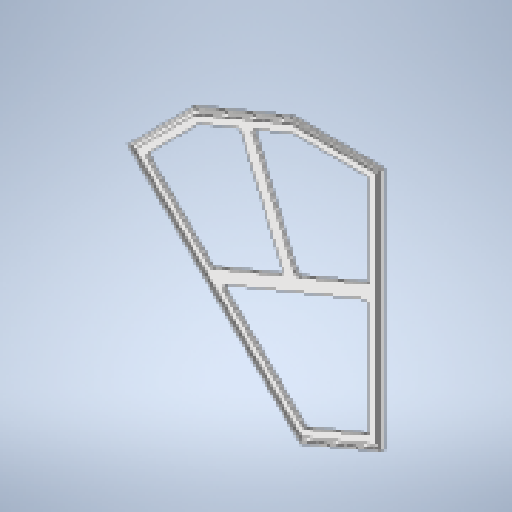
# Autodesk Inventor part: DMF 01 51 outside frame v2.1
Saved by Autodesk Inventor 2026.2 (Build 302298000, 298)
## iProperties
Created: 2024-05-05
Part Number: DMF 01 51 outside frame v2.1
Material: Generic
Document SubType Name: Modeling
Designer: pokla
Density: 1 g/cm^3
Appearance: Default
Author: pokla
Autodesk Inventor part; units mm, degrees
ref_plane "YZ Plane" through (0, 0, 0) normal (1, 0, 0) x (0, 1, 0)
ref_plane "XZ Plane" through (0, 0, 0) normal (0, 1, 0) x (-1, 0, 0)
ref_plane "XY Plane" through (0, 0, 0) normal (0, 0, 1) x (1, 0, 0)
sketch "Sketch1" plane through (0, 0, 0) normal (0, 0, 1) x (1, 0, 0)
  line L0 (0, 278.716) -> (197.082, 197.082) construction
  line L1 (197.082, 197.082) -> (278.716, 0) construction
  line L2 (278.716, 0) -> (197.082, -197.082) construction
  line L3 (197.082, -197.082) -> (0, -278.716) construction
  line L4 (0, -278.716) -> (-197.082, -197.082) construction
  line L5 (-197.082, -197.082) -> (-278.716, 0) construction
  line L6 (-278.716, 0) -> (-197.082, 197.082) construction
  line L7 (-197.082, 197.082) -> (0, 278.716)
  line L8 (-197.082, 197.082) -> (0, 278.716)
  line L9 (-461.6493, 774.8136) -> (-221.4406, 874.3113)
  line L10 (-98.541, 237.899) -> (-341.545, 824.5625) construction
  line L11 (-221.4406, 874.3113) -> (0, 874.3113)
  line L12 (0, 874.3113) -> (0, 278.716)
  line L13 (-461.6493, 774.8136) -> (-618.2315, 618.2315)
  line L14 (-618.2315, 618.2315) -> (-197.082, 197.082)
  point P0 (0, 0)
  point P1 (0, 0)
  dimension "d0" = 515
  dimension "d2" = 260
  dimension "d3" = 635
  constraints: 30 end point, 2 midpoint, 1 coincident, 1 horizontal, 1 parallel, 1 perpendicular, 1 symmetric about line, 1 vertical, 1 vertical alignment, 17 other
  measures "d0" distance between parallel lines of L5 L1
  measures "d2" distance of L9.start L9.end
  measures "d3" distance of L10.end L10.start
extrude "Extrusion1" add sketch "Sketch1" along normal mid plane 8
sketch "Sketch2" plane through (0, 0, 4) normal (0, 0, 1) x (1, 0, 0)
  line L0 (-221.4406, 874.3113) -> (-461.6493, 774.8136) projected
  line L1 (-461.6493, 774.8136) -> (-618.2315, 618.2315) projected
  line L2 (-236.7713, 532.4196) -> (-415.8262, 458.2526)
  line L3 (-197.082, 197.082) -> (0, 278.716) projected
  line L4 (-98.541, 237.899) -> (-341.545, 824.5625) construction
  line L5 (-618.2315, 618.2315) -> (-197.082, 197.082) projected
  line L6 (-415.8262, 458.2526) -> (-575.8051, 618.2315)
  line L7 (-575.8051, 618.2315) -> (-444.6557, 749.3809)
  line L8 (-444.6557, 749.3809) -> (-343.9227, 791.1058)
  line L9 (-236.7713, 532.4196) -> (-343.9227, 791.1058)
  line L10 (-209.0549, 543.9001) -> (-30, 618.067)
  line L11 (-30, 618.067) -> (-30, 844.3113)
  line L12 (-30, 844.3113) -> (-215.4733, 844.3113)
  line L13 (-215.4733, 844.3113) -> (-316.2063, 802.5863)
  line L14 (-209.0549, 543.9001) -> (-316.2063, 802.5863)
  line L15 (0, 278.716) -> (0, 874.3113) projected
  line L16 (-415.8262, 458.2526) -> (-30, 618.067) construction
  line L17 (-392.8652, 435.2916) -> (-30, 585.5953)
  line L18 (-190.043, 232.4694) -> (-30, 298.7614)
  line L19 (-30, 298.7614) -> (-30, 585.5953)
  line L20 (-190.043, 232.4694) -> (-392.8652, 435.2916)
  point P0 (0, 0)
  dimension "d11" = 30
  dimension "d12" = 280
  dimension "d13" = 30
  dimension "d14" = 30
  dimension "d15" = 15
  dimension "d21" = 30
  dimension "d22" = 30
  dimension "d23" = 30
  dimension "d24" = 30
  constraints: 32 end point, 5 parallel, 5 symmetric about line, 2 midpoint, 1 collinear
  measures "d11" distance between parallel lines of L5 L6
  measures "d12" distance between parallel lines of L8 L2
  measures "d13" distance between parallel lines of L0 L8
  measures "d14" distance between parallel lines of L1 L7
  measures "d15" distance between parallel lines of L9 L4
  measures "d21" distance between parallel lines of L16 L17
  measures "d22" distance between parallel lines of L5 L20
  measures "d23" distance between parallel lines of L19 L15
  measures "d24" distance between parallel lines of L18 L3
extrude "Extrusion2" cut sketch "Sketch2" against normal up to surface (8 mm away)
fillet "Fillet1" radius 10 12 edges at (-575.8051, 618.2315, 0) (-343.9227, 791.1058, 0) (-236.7713, 532.4196, 0) (-415.8262, 458.2526, 0) (-316.2063, 802.5863, 0) (-30, 844.3113, 0) (-30, 618.067, 0) (-209.0549, 543.9001, 0) (-392.8652, 435.2916, 0) (-30, 585.5953, 0) (-30, 298.7614, 0) (-190.043, 232.4694, 0)
sketch "Sketch4" plane through (0, 0, 4) normal (0, 0, 1) x (1, 0, 0)
  line L0 (-221.4406, 874.3113) -> (-461.6493, 774.8136) projected
  line L1 (0, 874.3113) -> (-221.4406, 874.3113) projected
  line L2 (-461.6493, 774.8136) -> (-618.2315, 618.2315) projected
  line L3 (-618.2315, 618.2315) -> (-197.082, 197.082) projected
  line L4 (-197.082, 197.082) -> (0, 278.716) projected
  line L5 (0, 278.716) -> (0, 874.3113) projected
  line L6 (-458.817, 770.5748) -> (-220.4461, 869.3113)
  line L7 (-220.4461, 869.3113) -> (-5, 869.3113)
  line L8 (-5, 869.3113) -> (-5, 282.0569)
  line L9 (-5, 282.0569) -> (-195.9088, 202.9799)
  line L10 (-195.9088, 202.9799) -> (-611.1604, 618.2315)
  line L11 (-611.1604, 618.2315) -> (-458.817, 770.5748)
  line L12 (-218.8548, 861.3113) -> (-454.2854, 763.7928)
  line L13 (-454.2854, 763.7928) -> (-599.8467, 618.2315)
  line L14 (-599.8467, 618.2315) -> (-194.0317, 212.4165)
  line L15 (-194.0317, 212.4165) -> (-13, 287.4023)
  line L16 (-13, 287.4023) -> (-13, 861.3113)
  line L17 (-13, 861.3113) -> (-218.8548, 861.3113)
  point P0 (0, 0)
  dimension "d26" = 5
  dimension "d27" = 8
  constraints: 24 end point, 10 other
  measures "d26" distance between parallel lines of L0 L6
  measures "d27" distance between parallel lines of L6 L12
extrude "Extrusion3" cut sketch "Sketch4" against normal blind 3 contours L6 L7 L8 L9 L10 L11
fillet "Fillet3" radius 16 2 edges at (-220.4461, 869.3113, 2.5) (-458.817, 770.5748, 2.5)
fillet "Fillet4" radius 8 2 edges at (-454.2854, 763.7928, 2.5) (-218.8548, 861.3113, 2.5)
equation "\"d0\" = Барабан_размер_по_плоскостям"
equation "\"d2\" = Кассета_длина_грани"
equation "\"d3\" = Кассета_высота"
equation "\"d11\" = d13"
equation "\"d14\" = d13"
equation "\"d15\" = 0.5 * d13"
equation "\"d21\" = d13"
equation "\"d22\" = d13"
equation "\"d23\" = d13"
equation "\"d24\" = d13"
equation "\"Барабан_размер_по_плоскостям\" = 515"
equation "\"Кассета_длина_грани\" = 260"
equation "\"Кассета_высота\" = 635"
body "Solid1"
